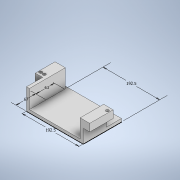
# Autodesk Inventor part: tttray
Saved by Autodesk Inventor 2020 (Build 240168000, 168)
## iProperties
Created: 2022-10-28
Part Number: tttray
Material: 일반
Document SubType Name: Modeling
Designer: SeungJin
Density: 1 g/cm^3
Appearance: 기본값
Author: SeungJin
Autodesk Inventor part; units mm, degrees
ref_plane "YZ Plane" through (0, 0, 0) normal (1, 0, 0) x (0, 1, 0)
ref_plane "XZ Plane" through (0, 0, 0) normal (0, 1, 0) x (-1, 0, 0)
ref_plane "XY Plane" through (0, 0, 0) normal (0, 0, 1) x (1, 0, 0)
sketch "스케치1" plane through (0, 0, 0) normal (0, 1, 0) x (-1, 0, 0)
  line L0 (96.25, 0) -> (-96.25, 0)
  line L1 (-96.25, 0) -> (-96.25, 67)
  line L2 (-96.25, 67) -> (96.25, 67)
  line L3 (96.25, 67) -> (96.25, 0)
  line L4 (96.25, 0) -> (-96.25, 0)
  line L5 (-96.25, 0) -> (-96.25, -63)
  line L6 (-96.25, -63) -> (96.25, -63)
  line L7 (96.25, -63) -> (96.25, 0)
  point P0 (0, 0)
  point P1 (0, 0)
  dimension "d0" = 192.5
  dimension "d1" = 67
  dimension "d2" = 192.5
  dimension "d3" = 63
  constraints: 16 end point, 4 parallel, 2 coincident, 2 horizontal, 2 perpendicular, 1 midpoint
  measures "d0" distance of L1.end L2.end
  measures "d1" distance of L2.end L0.start
  measures "d2" distance of L6.end L5.end
  measures "d3" distance of L6.end L0.start
extrude "돌출1" add sketch "스케치1" along normal blind 10
sketch "스케치2" plane through (0, 10, 0) normal (0, 1, 0) x (1, 0, 0)
  line L0 (-96.25, 0) -> (96.25, 0) projected
  line L1 (-96.25, -67) -> (96.25, -67) projected
  line L2 (86.25, -67) -> (86.25, 12.5)
  line L3 (96.25, -67) -> (96.25, 63) projected
  line L4 (96.25, 12.5) -> (86.25, 12.5)
  line L5 (-86.25, -67) -> (-86.25, 55)
  line L6 (-96.25, 63) -> (-96.25, -67) projected
  line L7 (-96.25, 55) -> (-86.25, 55)
  point P0 (0, 0)
  dimension "d6" = 10
  dimension "d7" = 12.5
  dimension "d8" = 10
  dimension "d9" = 55
  constraints: 8 end point, 4 point on line, 2 perpendicular, 2 vertical
  measures "d6" distance between parallel lines of L2 L3
  measures "d7" distance between parallel lines of L4 L0
  measures "d8" distance between parallel lines of L6 L5
  measures "d9" distance between parallel lines of L7 L0
extrude "돌출2" add sketch "스케치2" along normal blind 62 contours L6 L7 L5 L0 | L0 L5 L1 L6 | L2 L4 L3 L0 | L0 L3 L1 L2
sketch "스케치3" plane through (0, 72, 0) normal (0, 1, 0) x (1, 0, 0)
  line L0 (96.25, -67) -> (96.25, 12.5) projected
  line L1 (96.25, 12.5) -> (86.25, 12.5) projected
  line L2 (86.25, 12.5) -> (86.25, -67) projected
  line L3 (86.25, -67) -> (96.25, -67) projected
  line L4 (96.25, -67) -> (118.75, -67)
  line L5 (118.75, -67) -> (118.75, 12.5)
  line L6 (118.75, 12.5) -> (96.25, 12.5)
  line L7 (96.25, 12.5) -> (96.25, -67)
  point P0 (0, 0)
  dimension "d12" = 22.5
  constraints: 8 end point, 2 parallel, 1 horizontal, 1 perpendicular
  measures "d12" distance of L6.end L5.end
extrude "돌출3" add sketch "스케치3" against normal blind 25.3 contours L0 L6 L5 L4
sketch "스케치5" plane through (0, 72, 0) normal (0, 1, 0) x (1, 0, 0)
  line L0 (-96.25, 55) -> (-96.25, -67) projected
  line L1 (-96.25, -67) -> (-86.25, -67) projected
  line L2 (-86.25, -67) -> (-86.25, 55) projected
  line L3 (-86.25, 55) -> (-96.25, 55) projected
  line L4 (-96.25, 63) -> (-96.25, 55) projected
  line L5 (-96.25, 55) -> (-121.25, 55)
  line L6 (-121.25, 55) -> (-121.25, -12)
  line L7 (-121.25, -12) -> (-96.25, -12)
  line L8 (-96.25, -12) -> (-96.25, 55)
  line L9 (-96.25, 0) -> (96.25, 0) projected
  point P0 (0, 0)
  dimension "d15" = 25
  dimension "d16" = 12
  constraints: 8 end point, 2 parallel, 1 horizontal, 1 perpendicular
  measures "d15" distance between parallel lines of L6 L0
  measures "d16" distance between parallel lines of L9 L7
extrude "돌출4" add sketch "스케치5" against normal blind 23 contours L0 L7 L6 L5
sketch "스케치6" plane through (0, 72, 0) normal (0, 1, 0) x (1, 0, 0)
  line L0 (-96.25, 0) -> (96.25, 0) projected
  line L1 (86.25, 12.5) -> (86.25, -67) projected
  point P0 (0, 0)
  point P1 (111.25, 0)
  point P2 (-114.75, 0)
  point P3 (-102.75, 0)
  dimension "d19" = 25
  dimension "d20" = 214
  dimension "d21" = 12
  measures "d19" distance from line of point (111.25, 0) L1
  measures "d20" distance of point (-102.75, 0) point (111.25, 0)
  measures "d21" distance of point (-114.75, 0) point (-102.75, 0)
hole "구멍1" at (-114.75, 72, 0) at (-102.75, 72, 0) at (111.25, 72, 0) direction (0, -1, 0) diameter 5.5 end through all counterbore diameter 10 counterbore depth 15 clearance for "Socket Head Cap Screw ISO 4762" size "M5" standard "ISO"
